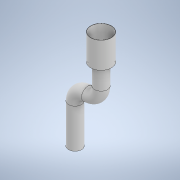
# Autodesk Inventor part: part12
Saved by Autodesk Inventor 2020 (Build 240168000, 168)
## iProperties
Created: 2019-08-01
Part Number: part12
Material: Generic
Document SubType Name: Modeling
Designer: ColinP
Density: 1 g/cm^3
Appearance: Default
Author: ColinP
Autodesk Inventor part; units mm, degrees
ref_plane "YZ Plane" through (0, 0, 0) normal (1, 0, 0) x (0, 1, 0)
ref_plane "XZ Plane" through (0, 0, 0) normal (0, 1, 0) x (-1, 0, 0)
ref_plane "XY Plane" through (0, 0, 0) normal (0, 0, 1) x (1, 0, 0)
sketch "Sketch5" plane through (0, 0, 0) normal (0, 0, 1) x (1, 0, 0)
  line L0 (0, 0) -> (0, 19.05)
  line L1 (0, 0) -> (0, 19.05)
  arc A0 (6.35, 25.4) -> (0, 19.05) centre (6.35, 19.05) ccw
  arc A1 (6.35, 25.4) -> (12.7, 31.75) centre (6.35, 31.75) ccw
  line L2 (12.7, 31.75) -> (12.7, 38.1)
  dimension "d17" = 19.05
  constraints: 6 end point, 4 point on circle, 2 centre point
  measures "d17" distance of L0.start L0.end
sketch "Sketch6" plane through (0, 0, 0) normal (0, 1, 0) x (-1, 0, 0)
  circle A0 centre (0, 0) radius 3.175
  circle A1 centre (0, 0) radius 3.048
  dimension "d23" = 6.35
  dimension "d24" = 6.096
  constraints: 2 centre point, 2 coincident
  measures "d23" diameter of A0
  measures "d24" diameter of A1
sweep "Sweep2" add profiles "Sketch6" path "Sketch5" path curves L0 A0
sketch "Sketch7" plane through (0, 0, 0) normal (0, 0, 1) x (1, 0, 0)
  line L0 (6.35, 22.225) -> (6.35, 28.575) projected
  arc A0 (6.35, 25.4) -> (12.7, 31.75) centre (6.35, 31.75) ccw
  point P0 (0, 0)
  constraints: 2 point on circle, 1 centre point, 1 midpoint
sketch "Sketch8" plane through (6.35, 25.4, 0) normal (1, 0, 0) x (0, 0, -1)
  circle A0 centre (0, 0) radius 3.175 projected
  circle A1 centre (0, 0) radius 3.048 projected
  point P0 (0, -25.4)
sweep "Sweep3" add profiles "Sketch8" path "Sketch7" separate body path curves A0
sketch "Sketch10" plane through (12.7, 31.75, 0) normal (0, 1, 0) x (1, 0, 0)
  circle A0 centre (0, 0) radius 3.048 projected
  circle A1 centre (0, 0) radius 3.175 projected
  point P0 (-12.7, 0)
extrude "Extrusion6" add sketch "Sketch10" along normal blind 10.16 bodies 2
sketch "Sketch11" plane through (12.7, 41.91, 0) normal (0, 1, 0) x (1, 0, 0)
  circle A0 centre (0, 0) radius 3.048 projected
  circle A1 centre (0, 0) radius 3.175 projected
  circle A2 centre (0, 0) radius 5.08
  circle A3 centre (0, 0) radius 4.953
  point P0 (-12.7, 0)
  dimension "d38" = 10.16
  dimension "d39" = 9.906
  constraints: 2 centre point, 2 coincident
  measures "d38" diameter of A2
  measures "d39" diameter of A3
extrude "Extrusion7" add sketch "Sketch11" along normal blind 1.27 contours A3 bodies 2
extrude "Extrusion8" add sketch "Sketch11" along normal blind 12.7 contours A2 bodies 2
body "Solid2"
body "Solid3"
